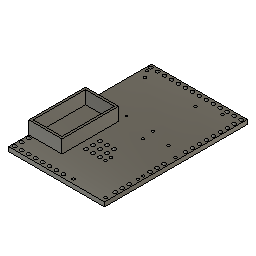
platte (Autodesk Fusion 360 design; units mm, degrees)
Autodesk Fusion 360 part; units mm, degrees
sketch "Skizze1" plane through (0, 0, 0) normal (0, 0, 1) x (1, 0, 0)
  line L0 (-55, 110) -> (55, 110)
  line L1 (55, 110) -> (55, -50)
  line L2 (55, -50) -> (-55, -50)
  line L3 (-55, -50) -> (-55, 110)
  circle A0 centre (0, 0) radius 2
  line L4 (0, 0) -> (-8, 0)
  line L5 (-8, 0) -> (-8, 8)
  line L6 (-8, 8) -> (0, 8)
  line L7 (0, 8) -> (0, 0)
  line L8 (-8, 8) -> (8, 8)
  line L9 (8, 8) -> (8, -8)
  line L10 (8, -8) -> (-8, -8)
  line L11 (-8, -8) -> (-8, 8)
  line L12 (0, 8) -> (8, 8)
  line L13 (8, 8) -> (8, -8)
  line L14 (8, -8) -> (0, -8)
  line L15 (0, -8) -> (0, 8)
  line L16 (-8, 0) -> (8, 0)
  line L17 (8, 0) -> (8, -8)
  line L18 (8, -8) -> (-8, -8)
  line L19 (-8, -8) -> (-8, 0)
  circle A1 centre (0, 8) radius 2
  circle A2 centre (-8, 8) radius 2
  circle A3 centre (-8, 0) radius 2
  circle A4 centre (-8, -8) radius 2
  circle A5 centre (0, -8) radius 2
  circle A6 centre (8, -8) radius 2
  circle A7 centre (8, 0) radius 2
  circle A8 centre (8, 8) radius 2
  circle A9 centre (-45.5, 97) radius 1.5
  circle A10 centre (12.5, 48) radius 1.5
  line L20 (-45.5, 97) -> (12.5, 97)
  line L21 (12.5, 97) -> (12.5, 48)
  line L22 (12.5, 48) -> (-45.5, 48)
  line L23 (-45.5, 48) -> (-45.5, 97)
  circle A11 centre (-45.5, 48) radius 1.5
  circle A12 centre (12.5, 97) radius 1.5
  line L24 (-50, 101.5) -> (35, 101.5)
  line L25 (35, 101.5) -> (35, 45.5)
  line L26 (35, 45.5) -> (-50, 45.5)
  line L27 (-50, 45.5) -> (-50, 101.5)
  line L28 (-45.5, 48) -> (12.5, 48)
  line L29 (12.5, 48) -> (12.5, 72.5)
  line L30 (-50, 45.5) -> (35, 45.5)
  line L31 (35, 45.5) -> (35, 73.5)
  line L32 (-51, 104.5) -> (36, 104.5)
  line L33 (36, 104.5) -> (36, 42.5)
  line L34 (36, 42.5) -> (-51, 42.5)
  line L35 (-51, 42.5) -> (-51, 104.5)
  circle A13 centre (-51, 42.5) radius 1.5
  circle A14 centre (-51, 104.5) radius 1.5
  circle A15 centre (36, 104.5) radius 1.5
  circle A16 centre (36, 42.5) radius 1.5
  line L36 (-7.5, 104.5) -> (-7.5, 42.5)
  line L37 (36, 73.5) -> (-51, 73.5)
  line L38 (-7.5, 101.5) -> (-7.5, 45.5)
  line L39 (35, 73.5) -> (-50, 73.5)
  line L40 (-52.5, 35.7098) -> (-19.5, 35.7098)
  line L41 (-19.5, 35.7098) -> (-19.5, -24.2902)
  line L42 (-19.5, -24.2902) -> (-52.5, -24.2902)
  line L43 (-52.5, -24.2902) -> (-52.5, 35.7098)
  line L44 (-36, 35.7098) -> (-36, -24.2902)
  line L45 (-19.5, 5.7098) -> (-52.5, 5.7098)
  line L46 (-55, 38.2098) -> (-17, 38.2098)
  line L47 (-17, 38.2098) -> (-17, -26.7902)
  line L48 (-17, -26.7902) -> (-55, -26.7902)
  line L49 (-55, -26.7902) -> (-55, 38.2098)
  line L50 (-36, 38.2098) -> (-36, -26.7902)
  line L51 (-17, 5.7098) -> (-55, 5.7098)
  line L52 (11.5, -5) -> (54.5, -5)
  line L53 (54.5, -5) -> (54.5, -48)
  line L54 (54.5, -48) -> (11.5, -48)
  line L55 (11.5, -48) -> (11.5, -5)
  line L56 (14.5, -8) -> (51.5, -8)
  line L57 (51.5, -8) -> (51.5, -45)
  line L58 (51.5, -45) -> (14.5, -45)
  line L59 (14.5, -45) -> (14.5, -8)
  circle A17 centre (14.5, -8) radius 1.5
  circle A18 centre (51.5, -8) radius 1.5
  circle A19 centre (51.5, -45) radius 1.5
  circle A20 centre (14.5, -45) radius 1.5
  line L60 (14.5, -26.5) -> (51.5, -26.5)
  line L61 (33, -8) -> (33, -45)
  line L62 (33, -5) -> (33, -48)
  line L63 (54.5, -26.5) -> (11.5, -26.5)
  line L64 (11.5, -5) -> (11.5, 38)
  circle A21 centre (14.5, -2) radius 1.5
  circle A22 centre (51.5, 35) radius 1.5
  circle A23 centre (14.5, 35) radius 1.5
  line L65 (11.5, 38) -> (54.5, 38)
  line L66 (33, 38) -> (33, -5)
  line L67 (54.5, 16.5) -> (11.5, 16.5)
  line L68 (33, 35) -> (33, -2)
  line L69 (14.5, 16.5) -> (51.5, 16.5)
  line L70 (14.5, 35) -> (51.5, 35)
  line L71 (54.5, -5) -> (11.5, -5)
  line L72 (51.5, 35) -> (51.5, -2)
  line L73 (54.5, 38) -> (54.5, -5)
  line L74 (51.5, -2) -> (14.5, -2)
  circle A24 centre (51.5, -2) radius 1.5
  line L75 (14.5, -2) -> (14.5, 35)
  line L76 (33, 16.5) -> (33, -26.5)
  line L77 (-55, 110) -> (55, 110)
  line L78 (55, 110) -> (55, 104.5)
  line L79 (55, 104.5) -> (-55, 104.5)
  line L80 (-55, 104.5) -> (-55, 110)
  line L81 (-55, 104.5) -> (-7.5, 104.5)
  line L82 (-7.5, 104.5) -> (-7.5, 73.5)
  line L83 (-7.5, 73.5) -> (-55, 73.5)
  line L84 (-55, 73.5) -> (-55, 104.5)
  line L85 (-55, 42.7098) -> (-36, 42.7098)
  line L86 (-36, 42.7098) -> (-36, 5.7098)
  line L87 (-36, 5.7098) -> (-55, 5.7098)
  line L88 (-55, 5.7098) -> (-55, 42.7098)
  line L89 (55, 42.5) -> (33, 42.5)
  line L90 (33, 42.5) -> (33, 16.5)
  line L91 (33, 16.5) -> (55, 16.5)
  line L92 (55, 16.5) -> (55, 42.5)
  line L93 (-55, 110) -> (55, 110)
  line L94 (55, 110) -> (55, 114)
  line L95 (55, 114) -> (-55, 114)
  line L96 (-55, 114) -> (-55, 110)
  circle A25 centre (-28, 110) radius 2
  circle A26 centre (-20, 110) radius 2
  circle A27 centre (-12, 110) radius 2
  circle A28 centre (-36, 110) radius 2
  circle A29 centre (-44, 110) radius 2
  circle A30 centre (-52, 110) radius 2
  circle A31 centre (-4, 110) radius 2
  circle A32 centre (4, 110) radius 2
  circle A33 centre (12, 110) radius 2
  circle A34 centre (20, 110) radius 2
  circle A35 centre (28, 110) radius 2
  circle A36 centre (36, 110) radius 2
  circle A37 centre (44, 110) radius 2
  circle A38 centre (52, 110) radius 2
  line L97 (52, 110) -> (52, 42.5)
  circle A39 centre (52, 102) radius 2
  circle A40 centre (52, 94) radius 2
  circle A41 centre (52, 86) radius 2
  circle A42 centre (52, 70) radius 2
  circle A43 centre (52, 78) radius 2
  circle A44 centre (52, 62) radius 2
  circle A45 centre (52, 54) radius 2
  circle A46 centre (52, 46) radius 2
  line L98 (-55, -50) -> (11.5, -50)
  line L99 (11.5, -50) -> (11.5, -46)
  line L100 (11.5, -46) -> (-55, -46)
  line L101 (-55, -46) -> (-55, -50)
  circle A47 centre (-52, -46) radius 2
  circle A48 centre (-44, -46) radius 2
  circle A49 centre (-36, -46) radius 2
  circle A50 centre (-28, -46) radius 2
  circle A51 centre (-20, -46) radius 2
  circle A52 centre (-12, -46) radius 2
  circle A53 centre (-4, -46) radius 2
  circle A54 centre (4, -46) radius 2
  circle A55 centre (-17.5, 48) radius 1
  line L102 (-52, -46) -> (-52, -24.2902)
  circle A56 centre (-52, -38) radius 2
  circle A57 centre (-52, -30) radius 2
  circle A58 centre (51.5, 22) radius 2
  circle A59 centre (51.5, 14) radius 2
  circle A60 centre (51.5, 6) radius 2
  circle A61 centre (51.5, -18) radius 2
  circle A62 centre (51.5, -26) radius 2
  circle A63 centre (51.5, -34) radius 2
  point P0 (-7.5, 73.5)
  point P1 (-7.5, 73.5)
  point P2 (-36, 5.7098)
  point P3 (-36, 5.7098)
  point P4 (33, -26.5)
  point P5 (33, -26.5)
  point P6 (33, 16.5)
  point P7 (33, 16.5)
  point P8 (-52, 110)
  point P9 (-44, 110)
  point P10 (-36, 110)
  dimension "d1" = 110
  dimension "d2" = 160
  dimension "d3" = 55
  dimension "d4" = 50
  dimension "d5" = 4
  dimension "d6" = 8
  dimension "d7" = 8
  dimension "d8" = 16
  dimension "d9" = 16
  dimension "d10" = 4
  dimension "d11" = 4
  dimension "d12" = 4
  dimension "d13" = 4
  dimension "d14" = 4
  dimension "d15" = 4
  dimension "d16" = 4
  dimension "d17" = 4
  dimension "d20" = 3
  dimension "d23" = 3
  dimension "d28" = 3
  dimension "d29" = 3
  dimension "d30" = 58
  dimension "d31" = 49
  dimension "d32" = 85
  dimension "d33" = 56
  dimension "d35" = 4.5
  dimension "d36" = 4.5
  dimension "d37" = 87
  dimension "d38" = 62
  dimension "d39" = 3
  dimension "d40" = 3
  dimension "d41" = 3
  dimension "d42" = 3
  dimension "d45" = 33
  dimension "d46" = 60
  dimension "d47" = 38
  dimension "d48" = 65
  dimension "d51" = 43
  dimension "d52" = 43
  dimension "d53" = 37
  dimension "d54" = 37
  dimension "d55" = 3
  dimension "d56" = 3
  dimension "d57" = 3
  dimension "d58" = 3
  dimension "d59" = 43
  dimension "d60" = 43
  dimension "d61" = 37
  dimension "d62" = 37
  dimension "d63" = 3
  dimension "d64" = 3
  dimension "d65" = 3
  dimension "d66" = 3
  dimension "d67" = 43
  dimension "d68" = 5.5
  dimension "d69" = 47.5
  dimension "d70" = 31
  dimension "d71" = 19
  dimension "d72" = 37
  dimension "d73" = 22
  dimension "d74" = 26
  dimension "d75" = 4
  dimension "d76" = 3
  dimension "d77" = 8
  dimension "d78" = 8
  dimension "d79" = 4
  dimension "d80" = 4
  dimension "d81" = 4
  dimension "d82" = 8
  dimension "d83" = 8
  dimension "d84" = 8
  dimension "d85" = 4
  dimension "d86" = 4
  dimension "d87" = 4
  dimension "d88" = 4
  dimension "d89" = 4
  dimension "d90" = 4
  dimension "d91" = 4
  dimension "d92" = 8
  dimension "d93" = 8
  dimension "d94" = 8
  dimension "d95" = 8
  dimension "d96" = 4
  dimension "d97" = 4
  dimension "d98" = 4
  dimension "d99" = 4
  dimension "d100" = 8
  dimension "d101" = 8
  dimension "d102" = 8
  dimension "d103" = 8
  dimension "d104" = 4
  dimension "d105" = 4
  dimension "d106" = 4
  dimension "d107" = 4
  dimension "d108" = 4
  dimension "d110" = 4
  dimension "d111" = 4
  dimension "d112" = 8
  dimension "d113" = 8
  dimension "d114" = 8
  dimension "d116" = 8
  dimension "d117" = 8
  dimension "d118" = 8
  dimension "d119" = 8
  dimension "d120" = 4
  dimension "d121" = 8
  dimension "d122" = 4
  dimension "d123" = 4
  dimension "d124" = 4
  dimension "d125" = 4
  dimension "d126" = 4
  dimension "d127" = 3
  dimension "d128" = 8
  dimension "d129" = 8
  dimension "d130" = 8
  dimension "d131" = 4
  dimension "d132" = 4
  dimension "d133" = 4
  dimension "d134" = 8
  dimension "d135" = 8
  dimension "d136" = 8
  dimension "d137" = 4
  dimension "d138" = 8
  dimension "d139" = 2
  dimension "d140" = 28
  dimension "d141" = 4
  dimension "d142" = 4
  dimension "d143" = 8
  dimension "d144" = 8
  dimension "d145" = 4
  dimension "d146" = 24
  dimension "d147" = 4
  dimension "d148" = 8
  dimension "d149" = 4
  dimension "d150" = 8
  dimension "d151" = 4
  dimension "d152" = 4
  dimension "d153" = 4
  dimension "d154" = 24
  dimension "d155" = 8
  dimension "d156" = 8
  constraint horizontal L0
  constraint vertical L1
  constraint horizontal L2
  constraint vertical L3
  constraint coincident A0.centre L4.start
  constraint horizontal L4
  constraint vertical L5
  constraint horizontal L6
  constraint vertical L7
  constraint horizontal L8
  constraint vertical L9
  constraint horizontal L10
  constraint vertical L11
  constraint horizontal L12
  constraint vertical L13
  constraint horizontal L14
  constraint vertical L15
  constraint horizontal L16
  constraint vertical L17
  constraint horizontal L18
  constraint vertical L19
  constraint coincident L6.end L7.start
  constraint coincident L5.end L6.start
  constraint coincident L4.end L5.start
  constraint coincident L10.end L11.start
  constraint coincident L14.end L15.start
  constraint coincident L9.end L10.start
  constraint coincident L16.end L17.start
  constraint coincident L8.end L9.start
  constraint horizontal L20
  constraint vertical L21
  constraint horizontal L22
  constraint vertical L23
  constraint coincident A10.centre L21.end
  constraint coincident A9.centre L20.start
  constraint coincident L22.end L23.start
  constraint coincident L20.end L21.start
  constraint horizontal L24
  constraint vertical L25
  constraint horizontal L26
  constraint vertical L27
  constraint horizontal L28
  constraint vertical L29
  constraint midpoint L21 L29.end
  constraint horizontal L30
  constraint vertical L31
  constraint midpoint L25 L31.end
  constraint horizontal L32
  constraint vertical L33
  constraint horizontal L34
  constraint vertical L35
  constraint coincident L34.end L35.start
  constraint coincident L32.start L35.end
  constraint coincident L32.end L33.start
  constraint coincident L33.end L34.start
  constraint midpoint L32 L36.start
  constraint midpoint L34 L36.end
  constraint midpoint L33 L37.start
  constraint midpoint L35 L37.end
  constraint midpoint L24 L38.start
  constraint midpoint L26 L38.end
  constraint midpoint L27 L39.end
  constraint midpoint L36 P1
  constraint midpoint L38 P1
  constraint coincident P1 P0
  constraint horizontal L40
  constraint vertical L41
  constraint horizontal L42
  constraint vertical L43
  constraint midpoint L40 L44.start
  constraint midpoint L42 L44.end
  constraint midpoint L41 L45.start
  constraint midpoint L43 L45.end
  constraint horizontal L46
  constraint vertical L47
  constraint horizontal L48
  constraint vertical L49
  constraint midpoint L46 L50.start
  constraint midpoint L48 L50.end
  constraint midpoint L47 L51.start
  constraint midpoint L49 L51.end
  constraint midpoint L50 P3
  constraint midpoint L44 P3
  constraint coincident P3 P2
  constraint horizontal L52
  constraint vertical L53
  constraint horizontal L54
  constraint vertical L55
  constraint horizontal L56
  constraint vertical L57
  constraint horizontal L58
  constraint vertical L59
  constraint coincident L56.start L59.end
  constraint coincident L56.end L57.start
  constraint coincident L57.end L58.start
  constraint coincident L58.end L59.start
  constraint midpoint L59 L60.start
  constraint midpoint L57 L60.end
  constraint midpoint L56 L61.start
  constraint midpoint L58 L61.end
  constraint midpoint L52 L62.start
  constraint midpoint L54 L62.end
  constraint midpoint L53 L63.start
  constraint midpoint L55 L63.end
  constraint midpoint L63 P5
  constraint midpoint L60 P5
  constraint coincident P5 P4
  constraint horizontal L65
  constraint vertical L73
  constraint horizontal L71
  constraint vertical L64
  constraint horizontal L70
  constraint vertical L72
  constraint horizontal L74
  constraint vertical L75
  constraint coincident A23.centre L70.start
  constraint coincident A22.centre L70.end
  constraint coincident L72.end L74.start
  constraint coincident A21.centre L74.end
  constraint midpoint L69.start L75
  constraint midpoint L69.end L72
  constraint midpoint L68.start L70
  constraint midpoint L68.end L74
  constraint midpoint L66.start L65
  constraint midpoint L62.start L71
  constraint midpoint L67.start L73
  constraint midpoint L67.end L64
  constraint midpoint P7 L67
  constraint midpoint P7 L69
  constraint coincident P7 P6
  constraint vertical L76
  constraint horizontal L77
  constraint vertical L78
  constraint horizontal L79
  constraint vertical L80
  constraint coincident L1 L78.end
  constraint horizontal L81
  constraint vertical L82
  constraint horizontal L83
  constraint vertical L84
  constraint horizontal L85
  constraint vertical L86
  constraint horizontal L87
  constraint vertical L88
  constraint coincident L3 L85.start
  constraint horizontal L89
  constraint vertical L90
  constraint horizontal L91
  constraint vertical L92
  constraint coincident L1 L89.start
  constraint horizontal L93
  constraint vertical L94
  constraint horizontal L95
  constraint vertical L96
  constraint coincident L0 P8
  constraint coincident L77 P9
  constraint coincident L93 P10
  constraint coincident L93 A25.centre
  constraint coincident L93 A26.centre
  constraint coincident L0 A27.centre
  constraint coincident P10 A28.centre
  constraint coincident P9 A29.centre
  constraint coincident P8 A30.centre
  constraint coincident L0 A31.centre
  constraint coincident L0 A32.centre
  constraint coincident L0 A33.centre
  constraint coincident L0 A34.centre
  constraint coincident L93 A35.centre
  constraint coincident L93 A36.centre
  constraint coincident L93 A37.centre
  constraint coincident L93 A38.centre
  constraint coincident A38.centre L97.start
  constraint coincident L89 L97.end
  constraint perpendicular L89 L97
  constraint coincident L97 A39.centre
  constraint coincident L97 A40.centre
  constraint coincident L97 A41.centre
  constraint coincident L97 A42.centre
  constraint coincident L97 A43.centre
  constraint coincident L97 A44.centre
  constraint coincident L97 A45.centre
  constraint coincident L97 A46.centre
  constraint horizontal L98
  constraint vertical L99
  constraint horizontal L100
  constraint vertical L101
  constraint coincident L55 L99.end
  constraint coincident L100 A47.centre
  constraint coincident L100 A48.centre
  constraint coincident L100 A49.centre
  constraint coincident L100 A50.centre
  constraint coincident L100 A51.centre
  constraint coincident L100 A52.centre
  constraint coincident L100 A53.centre
  constraint coincident L100 A54.centre
  constraint coincident L22 A55.centre
  constraint coincident A47.centre L102.start
  constraint coincident L42 L102.end
  constraint perpendicular L42 L102
  constraint coincident L102 A56.centre
  constraint coincident L102 A57.centre
  constraint coincident L72 A58.centre
  constraint coincident L72 A59.centre
  constraint coincident L72 A60.centre
  constraint coincident L57 A61.centre
  constraint coincident L57 A62.centre
  constraint coincident L57 A63.centre
  measures "d1" distance of L0.start L0.end
  measures "d2" distance of L0.start L2.end
  measures "d3" distance of A0.centre L3
  measures "d4" distance of A0.centre L2
  measures "d5" diameter of A0
  measures "d6" distance of A0.centre L4.end
  measures "d7" distance of A0.centre L6.end
  measures "d8" distance of L5.end L8.end
  measures "d9" distance of L5.end L10.end
  measures "d10" diameter of A1
  measures "d11" diameter of A2
  measures "d12" diameter of A3
  measures "d13" diameter of A4
  measures "d14" diameter of A5
  measures "d15" diameter of A6
  measures "d16" diameter of A7
  measures "d17" diameter of A8
  measures "d20" diameter of A9
  measures "d23" diameter of A10
  measures "d28" diameter of A11
  measures "d29" diameter of A12
  measures "d30" distance of A9.centre L20.end
  measures "d31" distance of A9.centre L22.end
  measures "d32" distance of L24.start L24.end
  measures "d33" distance of L24.start L26.end
  measures "d35" distance of L23 L27
  measures "d36" distance of L20 L24
  measures "d37" distance of L32.start L32.end
  measures "d38" distance of L32.start L34.end
  measures "d39" diameter of A13
  measures "d40" diameter of A14
  measures "d41" diameter of A15
  measures "d42" diameter of A16
  measures "d45" distance of L40.start L40.end
  measures "d46" distance of L40.start L42.end
  measures "d47" distance of L46.start L46.end
  measures "d48" distance of L46.start L48.end
  measures "d51" distance of L52.start L52.end
  measures "d52" distance of L52.start L54.end
  measures "d53" distance of L56.start L56.end
  measures "d54" distance of L56.start L58.end
  measures "d55" diameter of A17
  measures "d56" diameter of A18
  measures "d57" diameter of A19
  measures "d58" diameter of A20
  measures "d59" distance of L65.end L64.end
  measures "d60" distance of L52.start L64.end
  measures "d61" distance of A22.centre A23.centre
  measures "d62" distance of A21.centre A23.centre
  measures "d63" diameter of A23
  measures "d64" diameter of A22
  measures "d65" diameter of A24
  measures "d66" diameter of A21
  measures "d67" distance of P7 P5
  measures "d68" distance of L0.start L79.end
  measures "d69" distance of L79.end L36.start
  measures "d70" distance of L79.end L83.end
  measures "d71" distance of L85.start L85.end
  measures "d72" distance of L85.start L51.end
  measures "d73" distance of L89.start L89.end
  measures "d74" distance of L89.start L91.end
  measures "d75" distance of L0.start L95.end
  measures "d76" distance of L96 P8
  measures "d77" distance of P8 P9
  measures "d78" distance of P9 P10
  measures "d79" diameter of A25
  measures "d80" diameter of A26
  measures "d81" diameter of A27
  measures "d82" distance of P10 A25.centre
  measures "d83" distance of A25.centre A26.centre
  measures "d84" distance of A26.centre A27.centre
  measures "d85" diameter of A28
  measures "d86" diameter of A29
  measures "d87" diameter of A30
  measures "d88" diameter of A31
  measures "d89" diameter of A32
  measures "d90" diameter of A33
  measures "d91" diameter of A34
  measures "d92" distance of A27.centre A31.centre
  measures "d93" distance of A31.centre A32.centre
  measures "d94" distance of A32.centre A33.centre
  measures "d95" distance of A33.centre A34.centre
  measures "d96" diameter of A35
  measures "d97" diameter of A36
  measures "d98" diameter of A37
  measures "d99" diameter of A38
  measures "d100" distance of A34.centre A35.centre
  measures "d101" distance of A35.centre A36.centre
  measures "d102" distance of A36.centre A37.centre
  measures "d103" distance of A37.centre A38.centre
  measures "d104" diameter of A39
  measures "d105" diameter of A40
  measures "d106" diameter of A41
  measures "d107" diameter of A42
  measures "d108" diameter of A43
  measures "d110" diameter of A44
  measures "d111" diameter of A45
  measures "d112" distance of A38.centre A39.centre
  measures "d113" distance of A39.centre A40.centre
  measures "d114" distance of A40.centre A41.centre
  measures "d116" distance of A41.centre A43.centre
  measures "d117" distance of A42.centre A43.centre
  measures "d118" distance of A42.centre A44.centre
  measures "d119" distance of A44.centre A45.centre
  measures "d120" diameter of A46
  measures "d121" distance of A45.centre A46.centre
  measures "d122" distance of L2.end L100.end
  measures "d123" diameter of A47
  measures "d124" diameter of A48
  measures "d125" diameter of A49
  measures "d126" diameter of A50
  measures "d127" distance of L3 A47.centre
  measures "d128" distance of A47.centre A48.centre
  measures "d129" distance of A48.centre A49.centre
  measures "d130" distance of A49.centre A50.centre
  measures "d131" diameter of A51
  measures "d132" diameter of A52
  measures "d133" diameter of A53
  measures "d134" distance of A50.centre A51.centre
  measures "d135" distance of A51.centre A52.centre
  measures "d136" distance of A52.centre A53.centre
  measures "d137" diameter of A54
  measures "d138" distance of A53.centre A54.centre
  measures "d139" diameter of A55 L52.end
  measures "d140" distance of L22.end A55.centre
  measures "d141" diameter of A56
  measures "d142" diameter of A57
  measures "d143" distance of A47.centre A56.centre
  measures "d144" distance of A56.centre A57.centre
  measures "d145" diameter of A58
  measures "d146" vertical distance of A46.centre A58.centre
  measures "d147" diameter of A59
  measures "d148" distance of A58.centre A59.centre
  measures "d149" diameter of A60
  measures "d150" distance of A59.centre A60.centre
  measures "d151" diameter of A61
  measures "d152" diameter of A62
  measures "d153" diameter of A63
  measures "d154" distance of A60.centre A61.centre
  measures "d155" distance of A61.centre A62.centre
  measures "d156" distance of A62.centre A63.centre
extrude "Extrusion2" add sketch "Skizze1" along normal blind 5 contours L0 L77 L93 L94 L95 L96 A25 A26 A27 A28 A29 A30 A31 A32 A33 A34 A35 A36 A37 A38 | L0 L1 L77 L78 L79 L93 A38 L97 | L0 L3 L32 A14 A15 L77 L79 L80 L81 L93 A25 A26 A27 A28 A29 A30 A31 A32 A33 A34 A35 A36 A37 A38 L97 | L33 A15 A16 L79 L89 L97 A39 A40 A41 A42 A43 A44 A45 A46 | L1 L79 L89 L97 A39 A40 A41 A42 A43 A44 A45 A46 | L1 L34 A16 L65 L73 L89 L90 L91 L92 | L24 L25 L32 L33 A15 L36 L37 L79 L82 | L1 L2 L53 L54 L73 L91 L99 | L24 L27 L32 L35 A14 L36 L37 L79 L81 L82 L83 | L25 L26 L30 L31 L33 L34 A16 L36 L37 L89 | L52 L66 L67 L71 L72 L73 L74 A24 L76 L91 A59 A60 | A22 L65 L66 L67 L70 L72 L73 L90 L91 A58 | L3 L35 A14 L79 L81 L83 L84 | A9 L20 L23 L24 L27 L36 L37 L38 L39 L82 L83 | L20 L21 A12 L24 L25 L36 L37 L38 L39 L82 | A10 L21 L22 L25 L26 L28 L29 L30 L31 L36 L37 L38 L39 | L2 L3 L55 L98 L99 L100 L101 A47 A48 A49 A50 A51 A52 A53 A54 | L66 L67 L68 L69 L72 L74 A24 L76 L91 A59 A60 | A22 L66 L67 L68 L69 L70 L72 L90 L91 A58 | L52 L53 L56 L57 A18 L62 L63 L71 L76 A61 A62 | L3 L35 A13 L83 L85 | A9 L20 L23 L36 L37 L38 L39 L82 L83 | L20 L21 A12 L36 L37 L38 L39 L82 | A10 L21 L22 L28 L29 L36 L37 L38 L39 | L54 L55 L58 L59 A20 L62 L63 L99 | A23 L66 L67 L68 L69 L70 L75 L90 | A21 L66 L67 L68 L69 L74 L75 L76 | L64 A23 L65 L66 L67 L70 L75 L90 | L34 L46 L47 L48 L55 L64 L65 L86 L90 L100 A47 A48 A49 A50 A51 A52 A53 A54 L102 A56 A57 | L52 L55 L56 L59 A17 L62 L63 L71 L76 | L52 L64 A21 L66 L67 L71 L74 L75 L76 | L53 L54 L57 L58 A19 L62 L63 A62 A63 | L3 L34 A13 L46 L85 L86 L88 | L26 L27 L30 L34 L35 A13 L36 L37 L83 L85 L86 | L22 L23 A11 L26 L27 L28 L30 L36 L37 L38 L39 L83 A55 | L22 L23 A11 L28 L36 L37 L38 L39 L83 A55 | L3 L48 L100 A47 L102 A56 A57 | L56 L59 A17 L60 L61 L62 L63 L76 | L56 L57 A18 L60 L61 L62 L63 L76 A61 A62 | L3 L40 L43 L46 L49 L50 L51 L86 L87 L88 | L3 L42 L43 L48 L49 L51 L87 L102 | L57 L58 A19 L60 L61 L62 L63 A62 A63 | L58 L59 A20 L60 L61 L62 L63 | L34 A13 L85 L86 | L40 L41 L46 L47 L50 L51 L86 | L42 L48 L50 L102 | L42 L43 L44 L45 L50 L51 L87 | L40 L43 L44 L45 L50 L51 L86 L87 | L40 L41 L44 L45 L50 L51 L86 | L41 L42 L47 L48 L50 L51 | L41 L42 L44 L45 L50 L51 | A0 L9 L10 L13 L14 L15 L16 L17 L18 A5 A6 A7 | A0 L7 L8 L9 L12 L13 L15 L16 A1 A7 A8 | A0 L4 L5 L6 L7 L8 L11 L15 L16 A1 A2 A3 | A0 L4 L10 L11 L15 L16 L18 L19 A3 A4 A5
extrude "Extrusion3" add sketch "Skizze1" along normal blind 20 contours L3 L40 L43 L46 L49 L50 L51 L86 L87 L88 | L3 L42 L43 L48 L49 L51 L87 L102 | L40 L41 L46 L47 L50 L51 L86 | L42 L48 L50 L102 | L41 L42 L47 L48 L50 L51
